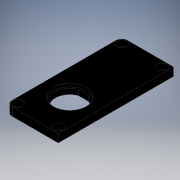
# Autodesk Inventor part: Connector Lid
Saved by Autodesk Inventor 2019 (Build 230136000, 136)
## iProperties
Created: 2016-08-11
Part Number: Connector Lid
Material: Aluminum 6061
Document SubType Name: Modeling
Designer: IEUser
Density: 2.7 g/cm^3
Appearance: Anodized - Black
Author: IEUser
Autodesk Inventor part; units mm, degrees
ref_plane "YZ Plane" through (0, 0, 0) normal (1, 0, 0) x (0, 1, 0)
ref_plane "XZ Plane" through (0, 0, 0) normal (0, 1, 0) x (-1, 0, 0)
ref_plane "XY Plane" through (0, 0, 0) normal (0, 0, 1) x (1, 0, 0)
sketch "Body Outline" plane through (0, 0, 0) normal (0, 1, 0) x (-1, 0, 0)
  line L0 (50, -22.5) -> (-50, -22.5)
  line L1 (-50, -22.5) -> (-50, 22.5)
  line L2 (-50, 22.5) -> (50, 22.5)
  line L3 (50, 22.5) -> (50, -22.5)
  point P0 (0, 0)
  dimension "d0" = 45
  dimension "d1" = 22.5
  dimension "d2" = 100
  dimension "d3" = 50
  constraints: 8 end point, 2 parallel, 1 horizontal, 1 perpendicular
  measures "d0" distance of L2.end L0.start
  measures "d1" distance from line of point (0, 0) L0
  measures "d2" distance of L0.start L0.end
  measures "d3" distance from line of point (0, 0) L3
extrude "Body" add sketch "Body Outline" along normal blind 7
sketch "Connector Hole Cross Section" plane through (0, 7, 0) normal (0, 1, 0) x (1, 0, 0)
  line L0 (-5.7, 4.4181) -> (-5.7, -4.4181)
  line L1 (-29.3, -4.4181) -> (-29.3, 4.4181)
  arc A0 (-5.7, 4.4181) -> (-29.3, 4.4181) centre (-17.5, 0) ccw
  arc A1 (-29.3, -4.4181) -> (-5.7, -4.4181) centre (-17.5, 0) ccw
  line L2 (50, 22.5) -> (-50, 22.5) projected
  line L3 (-50, 22.5) -> (-50, -22.5) projected
  point P0 (0, 0)
  dimension "d6" = 11.8
  dimension "d7" = 23.6
  dimension "d8" = 12.6
  dimension "d9" = 12.6
  dimension "d10" = 22.5
  dimension "d12" = 32.5
  constraints: 4 end point, 4 point on circle, 2 centre point, 1 parallel, 1 vertical
  measures "d6" distance from line of A0.centre L1
  measures "d7" distance between parallel lines of L0 L1
  measures "d8" radius of A0
  measures "d9" radius of A1
  measures "d10" distance from line of L2 A0.centre
  measures "d12" distance from line of L3 A0.centre
extrude "Connector Hole" cut sketch "Connector Hole Cross Section" along normal through all both and the other way through all
sketch "Connector Face Hole Cross Section" plane through (0, 7, 0) normal (0, 1, 0) x (1, 0, 0)
  circle A0 centre (-17.5, 0) radius 14.25
  line L0 (50, 22.5) -> (-50, 22.5) projected
  line L1 (-50, 22.5) -> (-50, -22.5) projected
  point P0 (0, 0)
  dimension "d15" = 22.5
  dimension "d16" = 32.5
  dimension "d17" = 28.5
  constraints: 1 centre point
  measures "d15" distance from line of L0 A0.centre
  measures "d16" distance from line of A0.centre L1
  measures "d17" diameter of A0
extrude "Connector Face Hole" cut sketch "Connector Face Hole Cross Section" against normal blind 2.5
fillet "Body Fillet" radius 5 2 edges at (-50, 3.5, -22.5) (50, 3.5, -22.5)
sketch "Lid Fastening Hole Pattern" plane through (0, 7, 0) normal (0, 1, 0) x (1, 0, 0)
  line L0 (-50, 17.5) -> (-50, -22.5) projected
  line L1 (45, 22.5) -> (-45, 22.5) projected
  point P0 (0, 0)
  point P1 (-45, 17.5)
  point P2 (45, 17.5)
  point P3 (-45, -17.5)
  point P4 (45, -17.5)
  dimension "d85" = 5
  dimension "d86" = 5
  dimension "d89" = 90
  dimension "d92" = 35
  constraints: 1 horizontal, 1 vertical, 3 other
  measures "d85" distance from line of point (-45, 17.5) L0
  measures "d86" distance from line of point (-45, 17.5) L1
  measures "d89" distance of point (-45, 17.5) point (45, 17.5)
  measures "d92" distance of point (-45, 17.5) point (-45, -17.5)
hole "Lid Fastening Holes" at (-45, 7, -17.5) at (45, 7, -17.5) at (-45, 7, 17.5) at (45, 7, 17.5) direction (0, -1, 0) diameter 5 end through all counterbore diameter 8.6 counterbore depth 5
equation "\"d1\" = 0.5 * d0"
equation "\"d3\" = 0.5 * d2"
equation "\"d6\" = 0.5 * d7"
equation "\"d9\" = d8"
equation "\"d10\" = 0.5 * d0"
equation "\"d15\" = 0.5 * d0"
equation "\"d85\" = d86"
body "Solid1"
